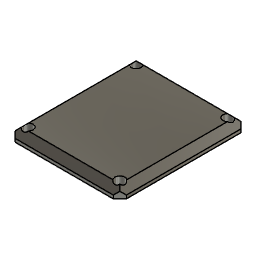
handle connector (Autodesk Fusion 360 design; units mm, degrees)
Autodesk Fusion 360 part; units mm, degrees
sketch "Sketch1" plane through (0, 0, 0) normal (0, 0, 1) x (1, 0, 0)
  line L0 (-17, 17.5) -> (-17, 0)
  line L1 (12, 14.5) -> (12, 0)
  line L2 (15, 19.5) -> (-15, 19.5)
  line L3 (-17, 0) -> (-12, 0)
  line L4 (-12, 14.5) -> (12, 14.5)
  line L5 (-12, 0) -> (-12, 14.5)
  line L6 (17, 17.5) -> (15, 19.5)
  circle A0 centre (-14, 16.5) radius 1.5
  circle A1 centre (14, 16.5) radius 1.5
  line L7 (-15, 19.5) -> (-17, 17.5)
  line L8 (17, 0) -> (17, 17.5)
  line L9 (12, 0) -> (17, 0)
  circle A2 centre (-14, -16.5) radius 1.5
  line L10 (12, -14.5) -> (12, 0)
  line L11 (-17, -17.5) -> (-17, 0)
  circle A3 centre (14, -16.5) radius 1.5
  line L12 (-17, 0) -> (-12, 0)
  line L13 (-12, -14.5) -> (12, -14.5)
  line L14 (15, -19.5) -> (-15, -19.5)
  line L15 (-15, -19.5) -> (-17, -17.5)
  line L16 (-12, 0) -> (-12, -14.5)
  line L17 (17, -17.5) -> (15, -19.5)
  line L18 (17, 0) -> (17, -17.5)
  line L19 (12, 0) -> (17, 0)
  constraint symmetric L0.end L9 L3.start
  constraint symmetric L2.end L9 L14.end
  constraint symmetric L3.end L9 L5.start
  constraint symmetric L1.start L9 L10.start
  constraint symmetric L4.start L9 L13.start
  constraint symmetric L1.end L9 L10.end
  constraint symmetric L8.start L9 L18.start
  constraint symmetric L6.start L9 L17.start
  constraint symmetric L2.start L9 L14.start
  constraint symmetric L0.start L9 L11.start
  constraint symmetric A0 L9 A2
  constraint symmetric A1 L9 A3
extrude "Extrude1" add sketch "Sketch1" along normal blind 3
chamfer "Chamfer1" distance 2 angle 45 4 edges at (-17, 0, 3) (0, -19.5, 3) (0, 19.5, 3) (17, 0, 3)
